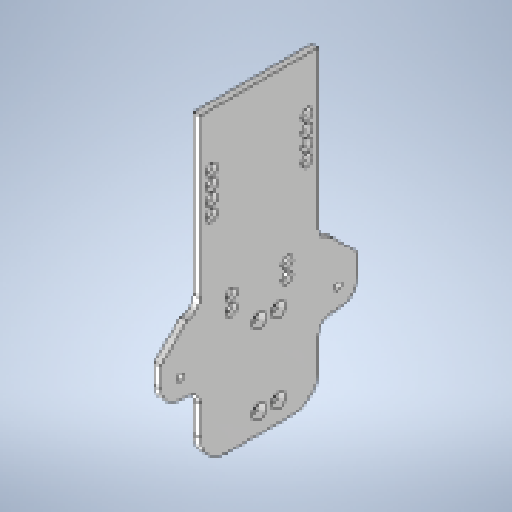
# Autodesk Inventor part: Bottom Plate
Saved by Autodesk Inventor 2023.2 (Build 272271000, 271)
## iProperties
Created: 2024-03-02
Part Number: Bottom Plate
Material: UHMW, White
Document SubType Name: Modeling
Designer: Nathan Cai
Mass: 30.5481 g
Surface Area: 231.408 cm^2
Volume: 32.4979 cm^3
Density: 0.94 g/cm^3
Appearance: Smooth - White
Author: Nathan Cai
Autodesk Inventor part; units mm, degrees
ref_plane "YZ Plane" through (0, 0, 0) normal (1, 0, 0) x (0, 1, 0)
ref_plane "XZ Plane" through (0, 0, 0) normal (0, 1, 0) x (-1, 0, 0)
ref_plane "XY Plane" through (0, 0, 0) normal (0, 0, 1) x (1, 0, 0)
sketch "Sketch1" plane through (0, 0, 0) normal (1, 0, 0) x (0, 1, 0)
  line L0 (-73.8187, -28.575) -> (73.8188, -28.575)
  line L1 (73.8188, -28.575) -> (73.8187, 28.575)
  line L2 (73.8187, 28.575) -> (-73.8188, 28.575)
  line L3 (-73.8188, 28.575) -> (-73.8187, -28.575)
  line L4 (-73.8187, -28.575) -> (73.8187, 28.575) construction
  line L5 (73.8188, -28.575) -> (-73.8188, 28.575) construction
  line L6 (-73.8187, 0) -> (73.8188, 0) construction
  line L7 (-8.7312, -47.625) -> (-40.4812, -47.625)
  line L8 (-40.4812, -47.625) -> (-40.4812, 47.625)
  line L9 (-40.4812, 47.625) -> (-8.7312, 47.625)
  line L10 (-8.7312, 47.625) -> (-8.7312, -47.625)
  line L11 (-8.7312, -47.625) -> (-40.4812, 47.625) construction
  line L12 (-40.4812, -47.625) -> (-8.7312, 47.625) construction
  circle A0 centre (-30.9563, 38.1) radius 9.525 construction
  circle A1 centre (-30.9563, 38.1) radius 1.7526
  circle A2 centre (-30.9563, -38.1) radius 1.7526
  line L13 (35.7188, 47.625) -> (73.8188, 47.625)
  line L14 (73.8188, 47.625) -> (73.8188, -47.625)
  line L15 (73.8188, -47.625) -> (35.7188, -47.625)
  line L16 (35.7188, -47.625) -> (35.7188, 47.625)
  line L17 (35.7188, 47.625) -> (73.8188, -47.625) construction
  line L18 (73.8188, 47.625) -> (35.7188, -47.625) construction
  line L19 (86.5188, -9.525) -> (61.1188, -9.525)
  line L20 (61.1188, -9.525) -> (61.1188, 9.525)
  line L21 (61.1188, 9.525) -> (86.5188, 9.525)
  line L22 (86.5188, 9.525) -> (86.5188, -9.525)
  line L23 (86.5188, -9.525) -> (61.1188, 9.525) construction
  line L24 (61.1188, -9.525) -> (86.5188, 9.525) construction
  point P0 (0, 0)
  point P1 (-24.6062, 0)
  point P2 (-8.7312, -28.575)
  point P3 (-40.4812, -28.575)
  point P4 (-40.4812, 28.575)
  point P5 (-8.7312, 28.575)
  point P6 (54.7687, 0)
  point P7 (35.7188, -28.575)
  point P8 (35.7187, 28.575)
  point P9 (73.8187, -9.525)
  point P10 (73.8187, 9.525)
  dimension "d0" = 147.6375
  dimension "d1" = 57.15
  dimension "d4" = 33.3375
  dimension "d5" = 31.75
  dimension "d6" = 19.05
  dimension "d7" = 3.5052
  dimension "d34" = 38.1
  dimension "d35" = 95.25
  dimension "d36" = 25.4
  dimension "d37" = 19.05
  constraints: 50 end point, 10 midpoint, 8 parallel, 4 horizontal, 4 perpendicular, 3 centre point, 3 point on line, 3 tangent, 1 coincident, 1 symmetric about line, 1 other
  measures "d0" distance of L2.end L1.end
  measures "d1" distance of L1.end L0.end
  measures "d4" distance between parallel lines of L3 L8
  measures "d5" distance between parallel lines of L8 L10
  measures "d6" distance between parallel lines of L2 L9
  measures "d7" diameter of A1
  measures "d34" distance of L14.end L15.end
  measures "d35" distance of L13.end L14.end
  measures "d36" distance of L20.end L21.end
  measures "d37" distance of L19.end L20.end
extrude "Extrusion1" add sketch "Sketch1" along normal blind 3.175 contours L3 L2 L8 L0 | L8 L2 L10 L0 | L0 L10 L7 L8 | L10 L2 L16 L0 | L8 L9 L10 L2 | L16 L2 L1 L21 L20 L19 L0 | L0 L14 L15 L16 | L16 L13 L14 L2
fillet "Fillet1" radius 9.525 2 edges at (1.5875, -40.4812, 47.625) (1.5875, -40.4812, -47.625)
fillet "Fillet2" radius 6.35 12 edges at (1.5875, -40.4812, 28.575) (1.5875, -40.4812, -28.575) (1.5875, -8.7312, -28.575) (1.5875, -8.7312, 28.575) (1.5875, 35.7188, -28.575) (1.5875, 35.7188, -47.625) (1.5875, 35.7188, 47.625) (1.5875, 35.7187, 28.575) (1.5875, 61.1188, 9.525) (1.5875, 73.8187, 9.525) (1.5875, 61.1188, -9.525) (1.5875, 73.8187, -9.525)
fillet "Fillet3" radius 12.7 2 edges at (1.5875, -73.8187, -28.575) (1.5875, -73.8188, 28.575)
chamfer "Chamfer3" distance 12.7 angle 45 2 edges at (1.5875, -8.7312, -47.625) (1.5875, -8.7312, 47.625)
sketch "Sketch2" plane through (3.175, 0, 0) normal (1, 0, 0) x (0, 0, -1)
  point P0 (-23.0187, 48.4188)
  point P1 (-23.0187, 42.0688)
  point P2 (-23.0187, 35.7188)
  point P3 (-23.0187, 29.3688)
  point P4 (23.0188, 48.4188)
  point P5 (23.0188, 42.0688)
  point P6 (23.0188, 35.7188)
  point P7 (23.0188, 29.3688)
  point P8 (13.4938, -8.7312)
  point P9 (13.4938, -15.0812)
  point P10 (-13.4937, -8.7312)
  point P11 (-13.4937, -15.0812)
hole "Hole1" at (3.175, 48.4188, 23.0187) at (3.175, 42.0688, 23.0187) at (3.175, 35.7188, 23.0187) at (3.175, 29.3688, 23.0187) at (3.175, 48.4188, -23.0188) at (3.175, 42.0688, -23.0188) at (3.175, 35.7188, -23.0188) at (3.175, 29.3688, -23.0188) at (3.175, -8.7312, -13.4938) at (3.175, -15.0812, -13.4938) at (3.175, -8.7312, 13.4937) at (3.175, -15.0812, 13.4937) direction (-1, 0, 0) diameter 3.2639 end through all countersink diameter 5.715 countersink angle 82
sketch "Sketch3" plane through (3.175, 0, 0) normal (1, 0, 0) x (0, 0, -1)
  point P0 (0, -26.1937)
  point P1 (9.525, -26.1937)
  point P2 (9.525, -64.2937)
  point P3 (0, -64.2937)
hole "Hole2" at (3.175, -26.1937, 0) at (3.175, -26.1937, -9.525) at (3.175, -64.2937, -9.525) at (3.175, -64.2937, 0) direction (-1, 0, 0) diameter 3.5052 end through all countersink diameter 7.0866 countersink angle 82
fillet "Fillet4" radius 1.5875 2 edges at (1.5875, 73.8188, 47.625) (1.5875, 73.8188, -47.625)
sketch "Sketch4" plane through (3.175, 0, 0) normal (1, 0, 0) x (0, 0, -1)
  point P0 (33.3375, 57.9438)
  point P1 (42.8625, 57.9438)
  point P2 (42.8625, 45.2438)
  point P3 (33.3375, 45.2438)
  point P4 (-42.8625, 45.2438)
  point P5 (-33.3375, 45.2438)
  point P6 (-33.3375, 57.9438)
  point P7 (-42.8625, 57.9438)
hole "Hole3" at (3.175, 57.9438, -33.3375) at (3.175, 57.9438, -42.8625) at (3.175, 45.2438, -42.8625) at (3.175, 45.2438, -33.3375) at (3.175, 45.2438, 42.8625) at (3.175, 45.2438, 33.3375) at (3.175, 57.9438, 33.3375) at (3.175, 57.9438, 42.8625) direction (-1, 0, 0) diameter 3.7973 end through all countersink diameter 7.0866 countersink angle 82
body "Solid1"
